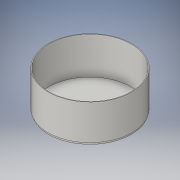
# Autodesk Inventor part: cover
Saved by Autodesk Inventor 2016 SP1 (Build 200210100, 210)
## iProperties
Created: 2015-12-11
Part Number: cover
Material: Acetal Resin, White
Document SubType Name: Modeling
Designer: ddeboer
Mass: 1322.68 g
Surface Area: 5844.94 cm^2
Volume: 928.194 cm^3
Density: 1.425 g/cm^3
Appearance: Smooth - White
Author: ddeboer
Autodesk Inventor part; units mm, degrees
ref_plane "YZ Plane" through (0, 0, 0) normal (1, 0, 0) x (0, 1, 0)
ref_plane "XZ Plane" through (0, 0, 0) normal (0, 1, 0) x (-1, 0, 0)
ref_plane "XY Plane" through (0, 0, 0) normal (0, 0, 1) x (1, 0, 0)
sketch "Sketch1" plane through (0, 0, 0) normal (0, 1, 0) x (-1, 0, 0)
  circle A0 centre (0, 0) radius 166.37
  dimension "d0" = 332.74
  constraints: 1 centre point, 1 coincident
  measures "d0" diameter of A0
extrude "Extrusion1" add sketch "Sketch1" along normal blind 152.4
sketch "Sketch2" plane through (0, 152.4, 0) normal (0, 1, 0) x (1, 0, 0)
  circle A0 centre (0, 0) radius 163.83
  dimension "d3" = 327.66
  constraints: 1 centre point, 1 coincident
  measures "d3" diameter of A0
extrude "Extrusion2" cut sketch "Sketch2" against normal blind 147.32
fillet "Fillet1" radius 12.7 1 edges at (166.37, 0, 0)
body "Solid1"
